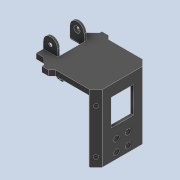
# Autodesk Inventor part: Z Axis Housing Frame Top Frunt
Saved by Autodesk Inventor 2022 (Build 260153000, 153)
## iProperties
Created: 2021-10-25
Part Number: Z Axis Housing Frame Top Frunt
Material: Generic
Document SubType Name: Modeling
Designer: Coy
Density: 1 g/cm^3
Appearance: Generic
Author: Coy
Autodesk Inventor part; units mm, degrees
sketch "Sketch1" plane through (0, 0, 0) normal (1, 0, 0) x (0, 1, 0)
  line L0 (0, 0) -> (105, 0)
  line L1 (105, 0) -> (105, 58)
  line L2 (105, 58) -> (0, 58)
  line L3 (0, 58) -> (0, 0)
  line L4 (40, 58) -> (40, 0) construction
  line L5 (30, 39) -> (10, 39) construction
  line L6 (10, 39) -> (10, 19) construction
  line L7 (10, 19) -> (30, 19) construction
  line L8 (30, 19) -> (30, 39) construction
  circle A0 centre (30, 39) radius 2.6
  circle A1 centre (30, 19) radius 2.6
  circle A2 centre (10, 19) radius 2.6
  circle A3 centre (10, 39) radius 2.6
  line L9 (95, 48) -> (50, 48)
  line L10 (50, 48) -> (50, 10)
  line L11 (50, 10) -> (95, 10)
  line L12 (95, 10) -> (95, 48)
  line L13 (105, 58) -> (0, 58)
  line L14 (0, 58) -> (0, 63)
  line L15 (0, 63) -> (105, 63)
  line L16 (105, 63) -> (105, 58)
  line L17 (105, 0) -> (0, 0)
  line L18 (0, 0) -> (0, -5)
  line L19 (0, -5) -> (105, -5)
  line L20 (105, -5) -> (105, 0)
  dimension "d0" = 58
  dimension "d1" = 105
  dimension "d2" = 40
  dimension "d3" = 20
  dimension "d4" = 20
  dimension "d5" = 10
  dimension "d6" = 19
  dimension "d7" = 5.2
  dimension "d8" = 5.2
  dimension "d9" = 5.2
  dimension "d10" = 5.2
  dimension "d11" = 10
  dimension "d12" = 10
  dimension "d13" = 10
  dimension "d14" = 10
  dimension "d31" = 5
  dimension "d32" = 5
  constraints: 42 end point, 10 parallel, 6 perpendicular, 5 horizontal, 4 centre point, 4 coincident, 3 point on line
  measures "d0" distance of L1.end L0.end
  measures "d1" distance of L1.end L2.end
  measures "d2" distance between parallel lines of L3 L4
  measures "d3" distance of L7.end L6.end
  measures "d4" distance of L6.end L5.end
  measures "d5" distance between parallel lines of L4 L8
  measures "d6" distance between parallel lines of L0 L7
  measures "d7" diameter of A0
  measures "d8" diameter of A1
  measures "d9" diameter of A2
  measures "d10" diameter of A3
  measures "d11" distance between parallel lines of L1 L12
  measures "d12" distance between parallel lines of L0 L11
  measures "d13" distance between parallel lines of L2 L9
  measures "d14" distance between parallel lines of L4 L10
  measures "d31" distance of L13.end L14.end
  measures "d32" distance of L18.end L17.end
extrude "Extrusion1" add sketch "Sketch1" along normal blind 5
sketch "Sketch4" plane through (0, 105, 63) normal (0, 1, 0) x (1, 0, 0)
  line L0 (0, 0) -> (0, 68) projected
  line L1 (0, 34) -> (-30.1174, 34) construction
  line L2 (5, 0) -> (5, 68) construction
  line L3 (5, 68) -> (-5.6066, 78.6066)
  line L4 (5, 68) -> (20, 68) construction
  line L5 (-5.6066, 78.6066) -> (-5.6066, 63)
  line L6 (-5.6066, 63) -> (0, 63)
  line L7 (5, 0) -> (-5.6066, -10.6066)
  line L8 (5, 0) -> (20, 0) construction
  line L9 (-5.6066, -10.6066) -> (-5.6066, 5)
  line L10 (-5.6066, 5) -> (0, 5)
  line L11 (5, 21.4) -> (0, 21.4) projected
  line L12 (5, 26.6) -> (0, 26.6) projected
  line L13 (0, 68) -> (0, 0) projected
  line L14 (0, 0) -> (5, 0) projected
  line L15 (5, 68) -> (5, 0) projected
  line L16 (0, 68) -> (5, 68) projected
  line L17 (-5.6066, 78.6066) -> (-7.1066, 78.6066)
  line L18 (-7.1066, 78.6066) -> (-7.1066, 63)
  line L19 (-7.1066, 63) -> (-5.6066, 63)
  line L20 (-5.6066, 63) -> (-5.6066, 78.6066)
  line L21 (-5.6066, 5) -> (-7.1066, 5)
  line L22 (-7.1066, 5) -> (-7.1066, -10.6066)
  line L23 (-7.1066, -10.6066) -> (-5.6066, -10.6066)
  line L24 (-5.6066, -10.6066) -> (-5.6066, 5)
  dimension "d40" = 15
  dimension "d41" = 135
  dimension "d42" = 5
  dimension "d123" = 1.5
  constraints: 34 end point, 5 parallel, 4 horizontal, 4 symmetric about line, 3 perpendicular, 2 point on line, 1 equal length, 1 midpoint
  measures "d40" distance of L2.end L3.end
  measures "d41" angle of L4 L3
  measures "d42" distance from line of L0.end L6
  measures "d123" distance of L19.end L18.end
extrude "Extrusion3" add sketch "Sketch4" against normal up to surface (105 mm away) contours L14 L7 L9 L10 L0 | L9 L23 L22 L21 | L6 L5 L3 L16 L0 | L19 L18 L17 L5
sketch "Sketch6" plane through (5, 0, 63) normal (0.7071068, 0, 0.7071068) x (0.7071068, 0, -0.7071068)
  line L0 (-15, 0) -> (0, 0) construction
  line L1 (-7.5, 0) -> (-7.5, 105) construction
  line L2 (-3.9645, 105) -> (-15, 105) construction
  circle A0 centre (-7.5, 90) radius 3.45
  circle A1 centre (-7.5, 15) radius 3.45
  point P0 (41.0122, 0)
  dimension "d52" = 6.9
  dimension "d53" = 6.9
  dimension "d54" = 15
  dimension "d55" = 15
  constraints: 3 point on line, 2 centre point, 2 end point, 1 midpoint, 1 vertical
  measures "d52" diameter of A0
  measures "d53" diameter of A1
  measures "d54" distance from line of L2 A0.centre
  measures "d55" distance from line of L0 A1.centre
extrude "Extrusion5" cut sketch "Sketch6" against normal blind 6
sketch "Sketch9" plane through (5, 0, 0) normal (1, 0, 0) x (0, 0, -1)
  circle A0 centre (-39, 30) radius 2.6 projected
  circle A1 centre (-39, 30) radius 4.75
  circle A2 centre (-19, 30) radius 2.6 projected
  circle A3 centre (-19, 30) radius 4.75
  circle A4 centre (-19, 10) radius 2.6 projected
  circle A5 centre (-19, 10) radius 4.75
  circle A6 centre (-39, 10) radius 2.6 projected
  circle A7 centre (-39, 10) radius 4.75
  point P0 (0, 0)
  dimension "d58" = 9.5
  dimension "d59" = 9.5
  dimension "d60" = 9.5
  dimension "d61" = 9.5
  constraints: 4 centre point, 4 coincident
  measures "d58" diameter of A1
  measures "d59" diameter of A7
  measures "d60" diameter of A3
  measures "d61" diameter of A5
extrude "Extrusion6" cut sketch "Sketch9" against normal blind 3
ref_plane "Work Plane2" through (0, 50, 29) normal (0, 0, 1) x (1, 0, 0)
mirror "Mirror2" about plane through (0, 50, 29) normal (0, 0, 1) of "Extrusion5"
ref_plane "Work Plane3" through (0, 114, 48) normal (0, 1, 0) x (1, 0, 0)
sketch "Sketch10" plane through (0, 114, 48) normal (0, 1, 0) x (1, 0, 0)
  line L0 (-5.6066, -25.6066) -> (-63.3066, -25.6066)
  line L1 (-5.6066, 63.6066) -> (-63.3066, 63.6066)
  line L2 (-63.3066, 63.6066) -> (-69.5, 69.8)
  line L3 (-63.3066, -25.6066) -> (-69.5, -31.8)
  line L4 (0, 48) -> (0, -10) construction
  line L5 (0, 19) -> (-80.5, 19) construction
  line L6 (-69.5, 69.8) -> (-80.5, 69.8)
  line L7 (-80.5, 19) -> (-80.5, 69.8)
  line L8 (5, 53) -> (-5.6066, 63.6066) construction
  line L9 (5, 53) -> (5, -15) construction
  line L10 (-5.6066, -25.6066) -> (5, -15) construction
  line L11 (-80.5, 69.6198) -> (-64.3701, 69.6198) construction
  line L12 (-64.3701, 69.6198) -> (-61.8569, 67.1066) construction
  line L13 (-61.8569, 67.1066) -> (-4.1569, 67.1066) construction
  line L14 (-4.1569, 67.1066) -> (8.5, 54.4497) construction
  line L15 (8.5, 54.4497) -> (8.5, -16.4497) construction
  line L16 (8.5, -16.4497) -> (-4.1569, -29.1066) construction
  line L17 (-4.1569, -29.1066) -> (-61.8569, -29.1066) construction
  line L18 (-61.8569, -29.1066) -> (-63.3449, -30.5947) construction
  line L19 (-5.6066, 63.6066) -> (-5.6066, 48) projected
  line L20 (-5.6066, 48) -> (-80.5, 48)
  line L21 (-5.6066, -10) -> (-5.6066, -25.6066) projected
  line L22 (-5.6066, -10) -> (-80.5, -10)
  line L23 (-80.5, -10) -> (-80.5, -74.1384)
  line L24 (-69.5, -31.8) -> (-80.5, -31.8)
  line L25 (0, 48) -> (0, -10) projected
  line L26 (-5.6066, -25.6066) -> (5, -15) projected
  line L27 (5, 53) -> (5, -15) projected
  line L28 (5, 53) -> (-5.6066, 63.6066) projected
  line L29 (-80.5, 19) -> (-80.5, -10)
  line L30 (0, -10) -> (-7.1066, -10) projected
  line L31 (-7.1066, -10) -> (-7.1066, -25.6066) projected
  line L32 (-7.1066, -25.6066) -> (-5.6066, -25.6066) projected
  line L33 (-5.6066, 63.6066) -> (-7.1066, 63.6066) projected
  line L34 (-7.1066, 63.6066) -> (-7.1066, 48) projected
  line L35 (-7.1066, 48) -> (0, 48) projected
  dimension "d69" = 135
  dimension "d70" = 135
  dimension "d71" = 80.5
  dimension "d72" = 3.5
  dimension "d75" = 80.5
  dimension "d81" = 11
  dimension "d82" = 11
  dimension "d83" = 101.6
  dimension "d84" = 50.8
  constraints: 40 end point, 5 horizontal, 4 perpendicular, 3 point on line, 1 midpoint, 6 other
  measures "d69" angle of L0 L3
  measures "d70" angle of L1 L2
  measures "d71" distance of L5.start L5.end
  measures "d72" distance between parallel lines of L8 L14
  measures "d75" distance between parallel lines of L4 L23
  measures "d81" distance of L6.end L2.end
  measures "d82" distance of L3.end L24.end
  measures "d83" distance of L6.end L24.end
  measures "d84" distance from line of L5 L24.end
extrude "Extrusion7" add sketch "Sketch10" against normal blind 9 contours L0 L31 L22 L21 | L21 L30 L25 L35 L19 L28 L27 L26 | L0 L3 L24 L23 L22 L31 | L19 L20 L34 L1 | L34 L20 L7 L6 L2 L1
sketch "Sketch12" plane through (-80.5, 114, 58) normal (-1, 0, 0) x (0, 0, 1)
  line L0 (-65.275, 0) -> (-49.75, 0)
  line L1 (-49.75, 0) -> (-49.75, -9)
  line L2 (-49.75, -9) -> (-65.275, -9)
  line L3 (-65.275, -9) -> (-65.275, 0)
  line L4 (7.275, 0) -> (-8.25, 0)
  line L5 (-8.25, 0) -> (-8.25, -9)
  line L6 (-8.25, -9) -> (7.275, -9)
  line L7 (7.275, -9) -> (7.275, 0)
  line L8 (-10, -19) -> (-48, -19) construction
  line L9 (-29, -19) -> (-29, -74.3121) construction
  line L10 (-79.8, 0) -> (-58, 0) construction
  point P0 (-58, -114)
  dimension "d85" = 15.525
  dimension "d86" = 9
  dimension "d87" = 15.525
  dimension "d88" = 9
  dimension "d89" = 41.5
  dimension "d90" = 20.75
  constraints: 18 end point, 4 parallel, 2 horizontal, 2 perpendicular, 1 collinear, 1 midpoint, 1 point on line, 1 vertical
  measures "d85" distance of L1.end L2.end
  measures "d86" distance of L0.end L1.end
  measures "d87" distance of L6.end L5.end
  measures "d88" distance of L5.end L4.end
  measures "d89" distance between parallel lines of L5 L1
  measures "d90" distance between parallel lines of L9 L5
extrude "Extrusion8" add sketch "Sketch12" along normal blind 24
chamfer "Chamfer2" distance 10.9 angle 45 2 edges at (-80.5, 109.5, -7.275) (-80.5, 109.5, 65.275)
sketch "Sketch13" plane through (0, 114, 48) normal (0, 1, 0) x (1, 0, 0)
  line L0 (-80.5, -1.75) -> (-80.5, -10) projected
  line L1 (-104.5, -1.75) -> (-104.5, -17.275) projected
  line L2 (-80.5, -1.75) -> (-104.5, -1.75)
  line L3 (-104.5, -1.75) -> (-104.5, -10)
  line L4 (-104.5, -10) -> (-80.5, -10)
  line L5 (-80.5, -10) -> (-80.5, -1.75)
  line L6 (-5.6066, -10) -> (-80.5, -10) projected
  line L7 (-80.5, 39.75) -> (-104.5, 39.75) projected
  line L8 (-104.5, 55.275) -> (-104.5, 39.75) projected
  line L9 (-80.5, 39.75) -> (-104.5, 39.75)
  line L10 (-104.5, 39.75) -> (-104.5, 48)
  line L11 (-104.5, 48) -> (-80.5, 48)
  line L12 (-80.5, 48) -> (-80.5, 39.75)
  line L13 (-80.5, 48) -> (-5.6066, 48) projected
  point P0 (0, 48)
  constraints: 16 end point, 4 parallel, 2 collinear, 2 horizontal, 2 perpendicular, 2 point on line
extrude "Extrusion9" add sketch "Sketch13" along normal blind 24
fillet "Fillet1" radius 12 4 edges at (-104.5, 138, 53.875) (-80.5, 138, 53.875) (-104.5, 138, 4.125) (-80.5, 138, 4.125)
sketch "Sketch14" plane through (-80.5, 114, 0) normal (0, 0, -1) x (-1, 0, 0)
  arc A0 (24, 12) -> (0, 12) centre (12, 12) ccw projected
  circle A1 centre (12, 12) radius 2.75
  point P0 (-80.5, -114)
  dimension "d101" = 5.5
  constraints: 1 centre point, 1 coincident
  measures "d101" diameter of A1
extrude "Extrusion10" cut sketch "Sketch14" against normal through all
sketch "Sketch15" plane through (0, 105, 48) normal (0, -1, 0) x (1, 0, 0)
  line L0 (-7.1066, 25.6066) -> (-63.3066, 25.6066) projected
  line L1 (-80.5, 10) -> (-5.6066, 10) projected
  line L2 (-63.3066, 25.6066) -> (-51.3066, 25.6066)
  line L3 (-51.3066, 25.6066) -> (-51.3066, 10)
  line L4 (-51.3066, 10) -> (-63.3066, 10)
  line L5 (-63.3066, 10) -> (-63.3066, 25.6066)
  point P0 (0, -48)
  point P1 (-5.6066, 25.6066)
  point P2 (-63.3066, 10)
  dimension "d104" = 12
  constraints: 8 end point, 2 parallel, 1 horizontal, 1 perpendicular, 1 point on line
  measures "d104" distance of L3.end L4.end
extrude "Extrusion11" add sketch "Sketch15" along normal blind 6
chamfer "Chamfer3" distance 3 distance2 6 1 edges at (-57.3066, 99, 73.6066) measured on face at (-55.3066, 99, 63.2022)
chamfer "Chamfer4" distance 3 distance2 6 1 edges at (-57.3066, 99, 58) measured on face at (-55.3066, 99, 62.2022)
fillet "Fillet3" radius 6 2 edges at (-63.3066, 99, 65.8033) (-51.3066, 99, 65.8033)
ref_plane "Work Plane4" through (0, 50, 29) normal (0, 0, 1) x (1, 0, 0)
mirror "Mirror3" about plane through (0, 50, 29) normal (0, 0, 1) of "Extrusion11", "Chamfer3", "Chamfer4", "Fillet3"
sketch "Sketch17" plane through (0, 0, 0) normal (-1, 0, 0) x (0, 0, 1)
  line L0 (0, 114) -> (0, 0) projected
  line L1 (0, 114) -> (58, 114)
  line L2 (58, 114) -> (58, 110.5)
  line L3 (58, 110.5) -> (0, 110.5)
  line L4 (0, 110.5) -> (0, 114)
  dimension "d120" = 3.5
  constraints: 8 end point, 2 parallel, 1 horizontal, 1 perpendicular
  measures "d120" distance of L1.end L2.end
extrude "Extrusion13" add sketch "Sketch17" along normal up to surface (80.5 mm away)
sketch "Sketch18" plane through (-63.3066, 114, 73.6066) normal (0, 0, 1) x (1, 0, 0)
  arc A0 (0, -9) -> (12, -9) centre (6, -9) ccw construction
  line L0 (0, -9) -> (12, -9) construction
  line L1 (12, -9) -> (12, -15) construction
  line L2 (12, -15) -> (0, -15) construction
  line L3 (0, -15) -> (0, -9) construction
  line L4 (5, -12.75) -> (7, -12.75)
  line L5 (7, -12.75) -> (7, -11.25)
  line L6 (7, -11.25) -> (5, -11.25)
  line L7 (5, -11.25) -> (5, -12.75)
  line L8 (5, -12) -> (0, -12) construction
  line L9 (6, -12.75) -> (6, -15) construction
  line L10 (6, -11.25) -> (6, -9) construction
  line L11 (7, -12) -> (12, -12) construction
  point P0 (63.3066, -114)
  dimension "d124" = 12
  dimension "d125" = 6
  dimension "d126" = 2
  dimension "d127" = 1.5
  constraints: 24 end point, 7 midpoint, 4 parallel, 4 perpendicular, 2 horizontal
  measures "d124" distance of L1.end L2.end
  measures "d125" distance of L0.end L1.end
  measures "d126" distance of L6.end L5.end
  measures "d127" distance of L5.end L4.end
extrude "Extrusion14" cut sketch "Sketch18" against normal through all
sketch "Sketch19" plane through (-104.5, 114, 58) normal (-1, 0, 0) x (0, 0, 1)
  line L0 (0, 0) -> (0, 12) projected
  line L1 (-8.25, 24) -> (0, 24) projected
  line L2 (0, 0) -> (-4.75, 0)
  line L3 (-4.75, 0) -> (-4.75, 24)
  line L4 (-4.75, 24) -> (0, 24)
  line L5 (0, 24) -> (0, 0)
  line L6 (-58, 0) -> (-58, 12) projected
  line L7 (-58, 24) -> (-49.75, 24) projected
  line L8 (-58, 0) -> (-53.25, 0)
  line L9 (-53.25, 0) -> (-53.25, 24)
  line L10 (-53.25, 24) -> (-58, 24)
  line L11 (-58, 24) -> (-58, 0)
  point P0 (-58, -114)
  dimension "d130" = 4.75
  dimension "d131" = 4.75
  constraints: 16 end point, 4 parallel, 2 horizontal, 2 perpendicular, 2 point on line
  measures "d130" distance of L3.end L4.end
  measures "d131" distance of L10.end L9.end
extrude "Extrusion15" cut sketch "Sketch19" against normal up to next
fillet "Fillet4" radius 3 2 edges at (-92.5, 105, 49.75) (-92.5, 105, 8.25)
chamfer "Chamfer5" distance 2.5 angle 45 2 edges at (-89.75, 126, 49.75) (-89.75, 126, 8.25)
equation "\"d5\" = -0.5 * d3 + 0.5 * d2"
equation "\"d6\" = -0.5 * d4 + 0.5 * d0"
equation "\"d8\" = d7"
equation "\"d9\" = d7"
equation "\"d10\" = d7"
equation "\"d12\" = d11"
equation "\"d13\" = d11"
equation "\"d14\" = d11"
equation "\"d53\" = d52"
equation "\"d59\" = d58"
equation "\"d60\" = d58"
equation "\"d61\" = d58"
equation "\"d75\" = d71"
equation "\"d82\" = d81"
equation "\"d84\" = 0.5 * d83"
equation "\"d87\" = d85"
equation "\"d90\" = 0.5 * d89"
body "Solid1"
